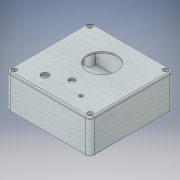
# Autodesk Inventor part: Box
Saved by Autodesk Inventor 2018.3 (Build 223284000, 284)
## iProperties
Created: 2018-06-03
Part Number: Box
Material: Generisch
Document SubType Name: Modeling
Designer: JochenAlt
Density: 1 g/cm^3
Appearance: Vorgabe
Author: JochenAlt
Autodesk Inventor part; units mm, degrees
ref_plane "YZ Plane" through (0, 0, 0) normal (1, 0, 0) x (0, 1, 0)
ref_plane "XZ Plane" through (0, 0, 0) normal (0, 1, 0) x (-1, 0, 0)
ref_plane "XY Plane" through (0, 0, 0) normal (0, 0, 1) x (1, 0, 0)
sketch "Skizze1" plane through (0, 0, 0) normal (0, 0, 1) x (1, 0, 0)
  line L0 (63, -70) -> (-63, -70)
  line L1 (-70, -63) -> (-70, 63)
  line L2 (-63, 70) -> (63, 70)
  line L3 (70, 63) -> (70, -63)
  line L4 (70, -70) -> (-70, 70) construction
  line L5 (-70, -70) -> (70, 70) construction
  arc A0 (70, 63) -> (63, 70) centre (63, 63) ccw
  line L6 (-63, 63) -> (63, 63) construction
  line L7 (63, 63) -> (63, -63) construction
  line L8 (63, -63) -> (-63, -63) construction
  line L9 (-63, -63) -> (-63, 63) construction
  circle A1 centre (-63, 63) radius 1.5
  circle A2 centre (63, 63) radius 1.5
  circle A3 centre (-63, -63) radius 1.5
  circle A4 centre (63, -63) radius 1.5
  circle A5 centre (-63, 63) radius 4
  circle A6 centre (63, 63) radius 4
  circle A7 centre (-63, -63) radius 4
  circle A8 centre (63, -63) radius 4
  line L10 (57.2554, 67) -> (-57.2554, 67)
  line L11 (-67, 57.2554) -> (-67, -57.2554)
  line L12 (-57.2554, -67) -> (57.2554, -67)
  line L13 (67, -57.2554) -> (67, 57.2554)
  arc A9 (-70, -63) -> (-63, -70) centre (-63, -63) ccw
  arc A10 (-57.2554, -67) -> (-67, -57.2554) centre (-63, -63) ccw
  arc A11 (67, -57.2554) -> (57.2554, -67) centre (63, -63) ccw
  arc A12 (57.2554, 67) -> (67, 57.2554) centre (63, 63) ccw
  arc A13 (-63, 70) -> (-70, 63) centre (-63, 63) ccw
  arc A14 (-67, 57.2554) -> (-57.2554, 67) centre (-63, 63) ccw
  line L14 (-67, 57.2554) -> (-67, 67) construction
  line L15 (-57.2554, 67) -> (-67, 67) construction
  line L16 (57.2554, 67) -> (67, 67) construction
  line L17 (67, 57.2554) -> (67, 67) construction
  line L18 (-67, -57.2554) -> (-67, -67) construction
  line L19 (-57.2554, -67) -> (-67, -67) construction
  line L20 (57.2554, -67) -> (67, -67) construction
  line L21 (67, -57.2554) -> (67, -67) construction
  line L22 (-61.1236, 66.25) -> (-59.2472, 63)
  line L23 (-59.2472, 63) -> (-61.1236, 59.75)
  line L24 (-61.1236, 59.75) -> (-64.8764, 59.75)
  line L25 (-64.8764, 59.75) -> (-66.7528, 63)
  line L26 (-66.7528, 63) -> (-64.8764, 66.25)
  line L27 (-64.8764, 66.25) -> (-61.1236, 66.25)
  line L28 (64.8764, 66.25) -> (66.7528, 63)
  line L29 (66.7528, 63) -> (64.8764, 59.75)
  line L30 (64.8764, 59.75) -> (61.1236, 59.75)
  line L31 (61.1236, 59.75) -> (59.2472, 63)
  line L32 (59.2472, 63) -> (61.1236, 66.25)
  line L33 (61.1236, 66.25) -> (64.8764, 66.25)
  line L34 (61.1236, -59.75) -> (64.8764, -59.75)
  line L35 (64.8764, -59.75) -> (66.7528, -63)
  line L36 (66.7528, -63) -> (64.8764, -66.25)
  line L37 (64.8764, -66.25) -> (61.1236, -66.25)
  line L38 (61.1236, -66.25) -> (59.2472, -63)
  line L39 (59.2472, -63) -> (61.1236, -59.75)
  line L40 (-59.2472, -63) -> (-61.1236, -66.25)
  line L41 (-61.1236, -66.25) -> (-64.8764, -66.25)
  line L42 (-64.8764, -66.25) -> (-66.7528, -63)
  line L43 (-66.7528, -63) -> (-64.8764, -59.75)
  line L44 (-64.8764, -59.75) -> (-61.1236, -59.75)
  line L45 (-61.1236, -59.75) -> (-59.2472, -63)
  arc A15 (63, -70) -> (70, -63) centre (63, -63) ccw
  point P0 (0, 0)
  dimension "d8" = 2
  dimension "d0" = 140
  dimension "d1" = 140
  dimension "d3" = 3
  dimension "d4" = 8
  dimension "d11" = 7
  dimension "d12" = 3
  dimension "d54" = 6.5
  constraints: 92 end point, 16 centre point, 16 coincident, 16 point on circle, 15 point on line, 12 equal radius, 11 perpendicular, 6 tangent, 5 equal length, 5 parallel, 3 horizontal, 2 midpoint, 1 collinear, 1 vertical, 52 other
  measures "d0" distance of L4.end L5.end
  measures "d1" distance of L5.end L4.start
  measures "d3" diameter of A1
  measures "d4" diameter of A5
  measures "d11" radius of A13
  measures "d12" distance between parallel lines of L10 L2
  measures "d54" distance between parallel lines of L24 L27
extrude "Extrusion1" add sketch "Skizze1" along normal blind 2 contours L0 A9 L1 A13 L2 A0 L3 A15 | A12 L13 A11 L12 A10 L11 A14 L10
extrude "Extrusion2" add sketch "Skizze1" along normal blind 2 from surface at 2 contours L0 A9 L1 A13 L2 A0 L3 A15 | A5 | A6 | A7 | A8 | A12 L13 A11 L12 A10 L11 A14 L10 | L22 L23 L24 L25 L26 L27 | L28 L29 L30 L31 L32 L33 | L34 L35 L36 L37 L38 L39 | L40 L41 L42 L43 L44 L45
extrude "Extrusion3" add sketch "Skizze1" along normal blind 50 from surface at 4 contours L0 A9 L1 A13 L2 A0 L3 A15 | A5 | A6 | A7 | A8 | L22 L23 L24 L25 L26 L27 | L28 L29 L30 L31 L32 L33 | L34 L35 L36 L37 L38 L39 | L40 L41 L42 L43 L44 L45
extrude "Extrusion4" add sketch "Skizze1" along normal blind 2 from surface at 54 separate body contours L0 A9 L1 A13 L2 A0 L3 A15 | A5 | A6 | A7 | A8 | A12 L13 A11 L12 A10 L11 A14 L10 | L22 L23 L24 L25 L26 L27 | L28 L29 L30 L31 L32 L33 | L34 L35 L36 L37 L38 L39 | L40 L41 L42 L43 L44 L45
extrude "Extrusion5" add sketch "Skizze1" along normal blind 2 from surface at 56 contours L0 A9 L1 A13 L2 A0 L3 A15 | A12 L13 A11 L12 A10 L11 A14 L10 bodies 2
extrude "Extrusion9" cut sketch "Skizze1" against normal blind 12 from surface at 54 contours L22 L23 L24 L25 L26 L27 | L28 L29 L30 L31 L32 L33 | L34 L35 L36 L37 L38 L39 | L40 L41 L42 L43 L44 L45 bodies 1
fillet "Rundung1" radius 2 7 edges at (70, 0, 0) (67.9497, 67.9497, 0) (0, 70, 0) (-67.9497, 67.9497, 0) (-70, 0, 0) (-67.9497, -67.9497, 0) (0, -70, 0)
fillet "Rundung2" radius 2 7 edges at (-67.9497, -67.9497, 58) (-70, 0, 58) (-67.9497, 67.9497, 58) (0, 70, 58) (67.9497, 67.9497, 58) (70, 0, 58) (0, -70, 58)
sketch "Skizze2" plane through (-63, 68, 58) normal (0, 0, 1) x (1, 0, 0)
  circle A0 centre (63, -48) radius 24.25
  circle A1 centre (63, -48) radius 25.5
  circle A2 centre (63, -98) radius 5
  circle A3 centre (63, -48) radius 28.5
  circle A4 centre (63, -48) radius 29
  circle A5 centre (33, -113) radius 6
  line L0 (63, 30) -> (63, -166) construction
  line L1 (-35, -68) -> (161, -68) construction
  circle A6 centre (93, -113) radius 3
  line L2 (33, -113) -> (93, -113) construction
  line L3 (33, -113) -> (63, -98) construction
  line L4 (63, -98) -> (93, -113) construction
  point P0 (63, -68)
  dimension "d22" = 48.5
  dimension "d28" = 51
  dimension "d29" = 20
  dimension "d30" = 10
  dimension "d31" = 50
  dimension "d63" = 3
  dimension "d68" = 0.5
  dimension "d91" = 12
  dimension "d92" = 6
  dimension "d96" = 60
  dimension "d97" = 15
  constraints: 7 centre point, 6 end point, 3 coincident, 2 point on line, 1 perpendicular, 1 symmetric about line
  measures "d22" diameter of A0
  measures "d28" diameter of A1
  measures "d29" distance of A0.centre point (63, -68)
  measures "d30" diameter of A2
  measures "d31" distance of L3.end A0.centre
  measures "d63" radial gap between concentric circles of A3 A1
  measures "d68" radial gap between concentric circles of A4 A3
  measures "d91" diameter of A5
  measures "d92" diameter of A6
  measures "d96" distance of L2.start L2.end
  measures "d97" distance from line of L2 L3.end
extrude "Extrusion6" cut sketch "Skizze2" against normal up to next contours A0 | A2 | A5 | A6 bodies 2
extrude "Extrusion7" cut sketch "Skizze2" along normal blind 2 from surface at -4 contours A1 bodies 2
sketch "Odroid" plane through (0, 0, 0) normal (0, 0, 1) x (1, 0, 0)
  line L0 (-59, -2.5) -> (-1, -2.5) construction
  line L1 (-1, -2.5) -> (-1, -51.5) construction
  line L2 (-1, -51.5) -> (-59, -51.5) construction
  line L3 (-59, -51.5) -> (-59, -2.5) construction
  circle A0 centre (-59, -2.5) radius 1.4
  circle A1 centre (-1, -2.5) radius 1.4
  circle A2 centre (-1, -51.5) radius 1.4
  circle A3 centre (-59, -51.5) radius 1.4
  line L4 (-60.5, 1) -> (20.5, 1)
  line L5 (22.5, -1) -> (22.5, -53)
  line L6 (20.5, -55) -> (-60.5, -55)
  line L7 (-62.5, -53) -> (-62.5, -1)
  line L8 (-62.5, 1) -> (22.5, -55) construction
  line L9 (-62.5, -55) -> (22.5, 1) construction
  line L10 (-59, -27) -> (-1, -27) construction
  arc A4 (-60.5, 1) -> (-62.5, -1) centre (-60.5, -1) ccw
  arc A5 (22.5, -1) -> (20.5, 1) centre (20.5, -1) ccw
  arc A6 (20.5, -55) -> (22.5, -53) centre (20.5, -53) ccw
  arc A7 (-62.5, -53) -> (-60.5, -55) centre (-60.5, -53) ccw
  circle A8 centre (-59, -51.5) radius 2.5
  circle A9 centre (-1, -51.5) radius 2.5
  circle A10 centre (-1, -2.5) radius 2.5
  circle A11 centre (-59, -2.5) radius 2.5
  line L11 (-54.5, 26.8133) -> (-0.5, 26.8133)
  line L12 (-0.5, 26.8133) -> (-0.5, 2.8133)
  line L13 (-0.5, 2.8133) -> (-54.5, 2.8133)
  line L14 (-54.5, 2.8133) -> (-54.5, 26.8133)
  circle A12 centre (-45.7, 24.3133) radius 2.5
  circle A13 centre (-9.3, 5.3133) radius 2.5
  circle A14 centre (-9.3, 5.3133) radius 1.4
  circle A15 centre (-45.7, 24.3133) radius 1.4
  line L15 (0.5, 26.8133) -> (54.5, 26.8133)
  line L16 (54.5, 26.8133) -> (54.5, 2.8133)
  line L17 (54.5, 2.8133) -> (0.5, 2.8133)
  line L18 (0.5, 2.8133) -> (0.5, 26.8133)
  circle A16 centre (9.3, 24.3133) radius 2.5
  circle A17 centre (45.7, 5.3133) radius 2.5
  circle A18 centre (45.7, 5.3133) radius 1.4
  circle A19 centre (9.3, 24.3133) radius 1.4
  line L19 (57.2554, 67) -> (-57.2554, 67) construction
  arc A20 (-67, 57.2554) -> (-57.2554, 67) centre (-63, 63) ccw construction
  line L20 (-67, 57.2554) -> (-67, -57.2554) construction
  arc A21 (-57.2554, -67) -> (-67, -57.2554) centre (-63, -63) ccw construction
  line L21 (-57.2554, -67) -> (57.2554, -67) construction
  arc A22 (67, -57.2554) -> (57.2554, -67) centre (63, -63) ccw construction
  line L22 (67, -57.2554) -> (67, 57.2554) construction
  arc A23 (57.2554, 67) -> (67, 57.2554) centre (63, 63) ccw construction
  line L23 (0, 93.9819) -> (0, -94.8915) construction
  line L24 (-94.9399, 0) -> (94.0768, 0) construction
  point P0 (0, 0)
  point P1 (-20, -27)
  point P2 (-20, -27)
  dimension "d32" = 58
  dimension "d33" = 49
  dimension "d34" = 2.8
  dimension "d35" = 56
  dimension "d36" = 85
  dimension "d37" = 3.5
  dimension "d38" = 27
  dimension "d39" = 20
  dimension "d40" = 2
  dimension "d41" = 5
  dimension "d47" = 24
  dimension "d49" = 2.5
  dimension "d50" = 2.5
  dimension "d51" = 8.8
  dimension "d53" = 8.8
  dimension "d73" = 24
  dimension "d74" = 2.5
  dimension "d75" = 2.5
  dimension "d76" = 8.8
  dimension "d77" = 8.8
  dimension "d78" = 1
  dimension "d87" = 54
  constraints: 38 end point, 20 centre point, 15 equal radius, 12 coincident, 9 point on line, 8 parallel, 8 point on circle, 8 tangent, 4 horizontal, 4 midpoint, 4 perpendicular, 2 collinear, 1 other
  measures "d32" distance of L0.start L0.end
  measures "d33" distance of L0.end L1.end
  measures "d34" diameter of A0
  measures "d35" distance of L9.end L8.end
  measures "d36" distance of L8.start L9.end
  measures "d37" distance between parallel lines of L3 L7
  measures "d38" vertical distance of point (-20, -27) point (0, 0)
  measures "d39" horizontal distance of point (-20, -27) point (0, 0)
  measures "d40" radius of A4
  measures "d41" diameter of A8
  measures "d47" distance of L11.end L12.end
  measures "d49" distance from line of L11 A12.centre
  measures "d50" distance from line of L13 A13.centre
  measures "d51" distance from line of A12.centre L14
  measures "d53" distance from line of L12 A13.centre
  measures "d73" distance of L16.start L16.end
  measures "d74" distance from line of L15 A16.centre
  measures "d75" distance from line of L17 A17.centre
  measures "d76" distance from line of A16.centre L18
  measures "d77" distance from line of L16 A17.centre
  measures "d78" distance between parallel lines of L18 L12
  measures "d87" distance of L11.start L11.end
extrude "Extrusion8" add sketch "Odroid" along normal blind 5 from surface at 4 contours A8 | A9 | A10 | A11 | A13 | A12 | A17 | A16 bodies 1
extrude "Extrusion11" add sketch "Skizze2" against normal blind 2 from surface at -4 separate body contours A1 | A3
extrude "Extrusion12" cut sketch "Skizze2" along normal blind 0.5 from surface at -4 contours A0 | A1 | A3 | A4 bodies 2
sketch "Skizze7" plane through (-63, 70, 54) normal (0, 1, 0) x (1, 0, 0)
  line L0 (126, 52) -> (126, 0) construction
  line L1 (0, 52) -> (126, 52) construction
  line L2 (0, 0) -> (0, 52) construction
  line L3 (0, 0) -> (126, 0) construction
  circle A0 centre (63, 30) radius 5
  line L4 (0, 52) -> (126, 52) construction
  line L5 (63, 52) -> (63, 0) construction
  line L6 (0, 0) -> (126, 0) construction
  circle A1 centre (63, 15) radius 3.5
  point P0 (63, 54)
  dimension "d80" = 10
  dimension "d81" = 30
  dimension "d83" = 7
  dimension "d84" = 15
  constraints: 2 centre point, 2 end point, 2 midpoint, 2 point on line
  measures "d80" diameter of A0
  measures "d81" distance from line of A0.centre L3
  measures "d83" diameter of A1
  measures "d84" distance of A1.centre A0.centre
extrude "Extrusion14" cut sketch "Skizze7" against normal up to surface (3 mm away) bodies 1
equation "\"d50\" = d49"
equation "\"d75\" = d74"
